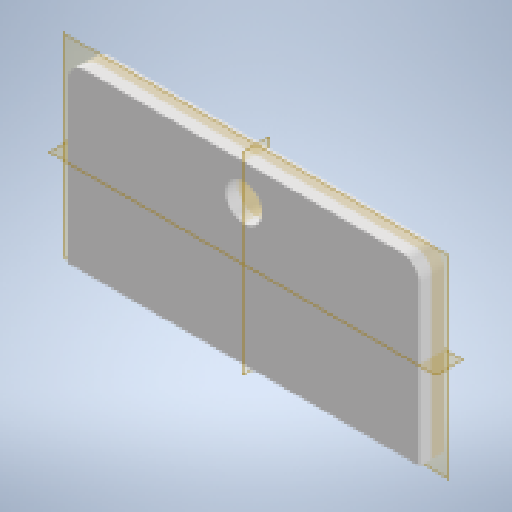
# Autodesk Inventor part: sessao_07_04_003_001
Saved by Autodesk Inventor 2026 (Build 300175000, 175)
## iProperties
Created: 2025-04-07
Part Number: sessao_07_04_003_001
Material: Generic
Document SubType Name: Modeling
Designer: Carlos Dias
Density: 1 g/cm^3
Appearance: Default
Author: Carlos Dias
Autodesk Inventor part; units mm, degrees
sketch "Sketch1" plane through (0, 0, 0) normal (0, 0, 1) x (1, 0, 0)
  line L0 (-50, 25) -> (50, 25)
  line L1 (50, 25) -> (50, -25)
  line L2 (50, -25) -> (-50, -25)
  line L3 (-50, -25) -> (-50, 25)
  line L4 (-50, 25) -> (50, -25) construction
  line L5 (50, 25) -> (-50, -25) construction
  circle A0 centre (0, 15) radius 5.2
  circle A1 centre (0, 15) radius 5 projected
  point P0 (0, 0)
  point P1 (0, 0)
  dimension "d0" = 100
  dimension "d1" = 50
  dimension "d2" = 15
  dimension "d7" = 10.4
  constraints: 12 end point, 2 midpoint, 2 parallel, 1 centre point, 1 coincident, 1 horizontal, 1 perpendicular, 1 vertical alignment
  measures "d0" distance of L0.start L0.end
  measures "d1" distance of L2.end L0.start
  measures "d2" distance of point (0, 0) A0.centre
  measures "d7" diameter of A0
extrude "Extrusion1" add sketch "Sketch1" along normal mid plane 7 contours L0 L1 L2 L3
fillet "Fillet1" radius 5 2 edges at (50, 25, 0) (-50, 25, 0)
chamfer "Chamfer1" distance 2 angle 45 1 edges at (-5.2, 15, 3.5)
body "Solid1"
